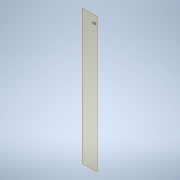
# Autodesk Inventor part: zaslepka_sruby-1
Saved by Autodesk Inventor 2022.3 (Build 263350000, 350)
## iProperties
Created: 2022-10-27
Part Number: zaslepka_sruby-1
Material: Generic
Document SubType Name: Modeling
Designer: komputer
Density: 1 g/cm^3
Appearance: Default
Author: komputer
Autodesk Inventor part; units mm, degrees
ref_plane "YZ Plane" through (0, 0, 0) normal (1, 0, 0) x (0, 1, 0)
ref_plane "XZ Plane" through (0, 0, 0) normal (0, 1, 0) x (-1, 0, 0)
ref_plane "XY Plane" through (0, 0, 0) normal (0, 0, 1) x (1, 0, 0)
ref_plane "Work Plane1" through (0, 0, 0) normal (0, 0, 1) x (1, 0, 0)
sketch "Sketch1" plane through (0, 0, 0) normal (0, 0, 1) x (1, 0, 0)
  line L0 (75, -675.6721) -> (75, 0) projected
  line L1 (0, 0) -> (75, 0) projected
  line L2 (0, -675.6721) -> (0, 0) projected
  line L3 (0, -675.6721) -> (75, -675.6721) projected
  arc A0 (57, -26) -> (57, -34) centre (57, -30) ccw projected
  line L4 (57, -26) -> (67, -26) projected
  arc A1 (67, -34) -> (67, -26) centre (67, -30) ccw projected
  line L5 (67, -34) -> (57, -34) projected
  arc A2 (57, -3.49) -> (57, -11.49) centre (57, -7.49) ccw projected
  line L6 (57, -3.49) -> (67, -3.49) projected
  arc A3 (67, -11.49) -> (67, -3.49) centre (67, -7.49) ccw projected
  line L7 (67, -11.49) -> (57, -11.49) projected
  line L8 (57, -7.49) -> (67, -7.49) construction
  line L9 (57, -11.2733) -> (67, -11.2733)
  line L10 (67, -3.7067) -> (57, -3.7067)
  arc A4 (57, -3.7067) -> (57, -11.2733) centre (57, -7.49) ccw
  arc A5 (67, -11.2733) -> (67, -3.7067) centre (67, -7.49) ccw
  point P0 (62, -7.49)
  constraints: 8 end point, 4 point on circle, 4 tangent, 2 centre point, 1 horizontal, 1 midpoint, 1 parallel
extrude "Extrusion1" add sketch "Sketch1" against normal blind 2.5 contours A4 L10 A5 L9
body "Solid1"
